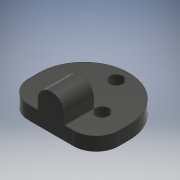
# Autodesk Inventor part: Support capteur
Saved by Autodesk Inventor 2017 (Build 210142000, 142)
## iProperties
Company: FABLAB Frenchmakers
Part Number: Support capteur
Project: 1420 VAUBAN 3D XL
Material: Plastique ABS
Catalog Web Link: http://www.frenchmakers.com/
Document SubType Name: Modeling
Designer: FABLAB Frenchmakers
Mass: 1.03914 g
Surface Area: 9.10518 cm^2
Volume: 0.980323 cm^3
Density: 1.06 g/cm^3
Appearance: Lisse - Noir
Stock Number: 1420-06-01
Autodesk Inventor part; units mm, degrees
ref_plane "YZ Plane" through (0, 0, 0) normal (1, 0, 0) x (0, 1, 0)
ref_plane "XZ Plane" through (0, 0, 0) normal (0, 1, 0) x (-1, 0, 0)
ref_plane "XY Plane" through (0, 0, 0) normal (0, 0, 1) x (1, 0, 0)
sketch "Esquisse1" plane through (0, 0, 0) normal (0, 0, 1) x (1, 0, 0)
  arc A0 (10, 7.25) -> (-10, 7.25) centre (0, 7.25) ccw
  line L0 (-10, 0) -> (10, 0)
  line L1 (10, 0) -> (10, 7.25)
  line L2 (-10, 7.25) -> (-10, 0)
  point P0 (0, 0)
  point P1 (0, 4.9938)
  point P2 (0, 0)
  dimension "d0" = 20
  dimension "d1" = 17.25
  constraints: 6 end point, 2 point on circle, 2 vertical alignment, 1 centre point, 1 coincident, 1 horizontal, 1 midpoint, 1 parallel, 1 perpendicular, 1 tangent
  measures "d0" diameter of A0
extrude "Extrusion1" add sketch "Esquisse1" along normal blind 3
fillet "Congé1" radius 5 2 edges at (-10, 0, 1.5) (10, 0, 1.5)
sketch "Esquisse2" plane through (-5, 0, 0) normal (0, -1, 0) x (1, 0, 0)
  line L0 (2, 3) -> (8, 3)
  line L1 (8, 3) -> (8, 5)
  line L2 (5, 8) -> (5, 8)
  line L3 (2, 5) -> (2, 3)
  line L4 (0, 0) -> (10, 0) projected
  line L5 (0, 3) -> (10, 3) projected
  arc A0 (5, 8) -> (2, 5) centre (5, 5) ccw
  arc A1 (8, 5) -> (5, 8) centre (5, 5) ccw
  point P0 (5, 0)
  point P1 (5, 3)
  point P2 (5, 0)
  dimension "d5" = 8
  dimension "d7" = 3
  dimension "d8" = 6
  constraints: 8 end point, 4 point on circle, 4 tangent, 2 centre point, 2 midpoint, 2 parallel, 1 collinear, 1 concentric, 1 horizontal, 1 perpendicular, 1 vertical alignment
  measures "d5" distance between parallel lines of L4 L2
  measures "d7" radius of A0
  measures "d8" distance between parallel lines of L1 L3
extrude "Extrusion2" add sketch "Esquisse2" against normal blind 6.5
sketch "Esquisse3" plane through (0, 0, 3) normal (0, 0, 1) x (1, 0, 0)
  line L0 (-3, 0) -> (3, 0) projected
  point P0 (0, 0)
  point P1 (-4.6, 6.75)
  point P2 (4.6, 6.75)
  point P3 (0, 14.5)
  point P4 (0, 0)
  dimension "d11" = 9.2
  dimension "d12" = 4.6
  dimension "d13" = 6.75
  dimension "d14" = 14.5
  constraints: 1 horizontal alignment, 1 midpoint, 1 vertical alignment
  measures "d11" distance of point (4.6, 6.75) point (-4.6, 6.75)
  measures "d12" horizontal distance of point (-4.6, 6.75) point (0, 0)
  measures "d13" distance from line of L0 point (-4.6, 6.75)
  measures "d14" distance from line of L0 point (0, 14.5)
hole "Perçage1" at (-4.6, 6.75, 3) at (4.6, 6.75, 3) at (0, 14.5, 3) direction (0, 0, -1) diameter 3 depth 8 tip angle 118
equation "\"d7\" = 0.5 * d8"
equation "\"d12\" = 0.5 * d11"
